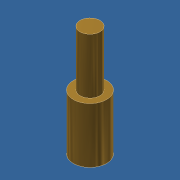
# Autodesk Inventor part: S1702_butee
Saved by Autodesk Inventor 2015 SP2 (Build 190223200, 223)
## iProperties
Created: 2017-10-31
Part Number: S1702_butee
Project: S1702_circuit_voiture
Material: CuZn36Pb3-HA laiton
Description: Butée
Document SubType Name: Modeling
Designer: Benoit.CURCHOD2
Authority: Ø4x10
Density: 8.5 g/cm^3
Appearance: Laiton - Satiné
Mass: 0.408564 g
Surface Area: 0.895354 cm^2
Volume: 0.0480664 cm^3
Material number: ---
Author: Benoit.CURCHOD2
Autodesk Inventor part; units mm, degrees
ref_plane "Plan YZ" through (0, 0, 0) normal (1, 0, 0) x (0, 1, 0)
ref_plane "Plan XZ" through (0, 0, 0) normal (0, 1, 0) x (-1, 0, 0)
ref_plane "Plan XY" through (0, 0, 0) normal (0, 0, 1) x (1, 0, 0)
sketch "Esquisse1" plane through (0, 0, 0) normal (0, 0, 1) x (1, 0, 0)
  circle A0 centre (0, 0) radius 1.5
  dimension "d0" = 3
  constraints: 1 centre point, 1 coincident
  measures "d0" diameter of A0
extrude "Extrusion1" add sketch "Esquisse1" along normal blind 10
sketch "Esquisse6" plane through (0, 0, 10) normal (0, 0, 1) x (1, 0, 0)
  circle A0 centre (0, 0) radius 0.9
  circle A1 centre (0, 0) radius 1.5 projected
  dimension "d6" = 1.8
  constraints: 1 centre point, 1 coincident
  measures "d6" diameter of A0
extrude "Extrusion2" cut sketch "Esquisse6" against normal blind 5
